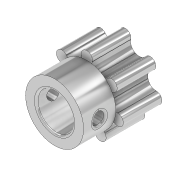
# Autodesk Inventor part: 4th Axis Drive Gears
Saved by Autodesk Inventor 2020 (Build 240168000, 168)
## iProperties
Created: 2021-06-27
Part Number: 4th Axis Drive Gears
Material: Generic
Document SubType Name: Modeling
Designer: Coy
Density: 1 g/cm^3
Appearance: Chrome - Polished
Author: Coy
Autodesk Inventor part; units mm, degrees
ref_plane "YZ Plane" through (0, 0, 0) normal (1, 0, 0) x (0, 1, 0)
ref_plane "XZ Plane" through (0, 0, 0) normal (0, 1, 0) x (-1, 0, 0)
ref_plane "XY Plane" through (0, 0, 0) normal (0, 0, 1) x (1, 0, 0)
sketch "Sketch1" plane through (0, 0, 0) normal (0, 0, 1) x (1, 0, 0)
  circle A0 centre (0, 0) radius 2.6
  circle A1 centre (0, 0) radius 6 construction
  line L0 (1.0268, 4.6361) -> (1.0416, 4.7025)
  line L1 (-1.0268, 4.6361) -> (-1.0416, 4.7025)
  line L2 (0, 0) -> (0, 12.6837) construction
  arc A2 (1.0416, 4.7025) -> (-1.0416, 4.7025) centre (0, 4.9332) ccw
  arc A3 (1.0268, 4.6361) -> (1.615, 3.4397) centre (2.0684, 4.4054) ccw
  arc A4 (-1.615, 3.4397) -> (-1.0268, 4.6361) centre (-2.0684, 4.4054) ccw
  arc A5 (-3.6962, 0.882) -> (-4.2649, 2.0877) centre (-4.7339, 1.1296) ccw
  arc A6 (-3.0272, 3.7463) -> (-4.326, 2.1176) centre (-3.8569, 3.0758) ccw
  arc A7 (-2.9844, 3.6934) -> (-1.6823, 3.4073) centre (-2.1546, 4.3639) ccw
  line L3 (-4.2649, 2.0877) -> (-4.326, 2.1176)
  line L4 (-2.9844, 3.6934) -> (-3.0272, 3.7463)
  arc A8 (-2.9941, -2.3399) -> (-4.2914, -2.0327) centre (-3.8347, -2.9968) ccw
  arc A9 (-4.8164, -0.031) -> (-4.3528, -2.0618) centre (-4.8095, -1.0977) ccw
  arc A10 (-4.7483, -0.0305) -> (-3.7129, 0.8091) centre (-4.7552, 1.0363) ccw
  line L5 (-4.2914, -2.0327) -> (-4.3528, -2.0618)
  line L6 (-4.7483, -0.0305) -> (-4.8164, -0.031)
  arc A11 (-0.0374, -3.7998) -> (-1.0864, -4.6225) centre (-0.0479, -4.8666) ccw
  arc A12 (-2.9788, -3.7849) -> (-1.1019, -4.6887) centre (-2.1404, -4.4447) ccw
  arc A13 (-2.9367, -3.7314) -> (-2.9475, -2.3984) centre (-3.775, -3.0717) ccw
  line L7 (-1.0864, -4.6225) -> (-1.1019, -4.6887)
  line L8 (-2.9367, -3.7314) -> (-2.9788, -3.7849)
  arc A14 (2.9475, -2.3984) -> (2.9367, -3.7314) centre (3.775, -3.0717) ccw
  arc A15 (1.1019, -4.6887) -> (2.9788, -3.7849) centre (2.1404, -4.4447) ccw
  arc A16 (1.0864, -4.6225) -> (0.0374, -3.7998) centre (0.0479, -4.8666) ccw
  line L9 (2.9367, -3.7314) -> (2.9788, -3.7849)
  line L10 (1.0864, -4.6225) -> (1.1019, -4.6887)
  arc A17 (3.7129, 0.8091) -> (4.7483, -0.0305) centre (4.7552, 1.0363) ccw
  arc A18 (4.3528, -2.0618) -> (4.8164, -0.031) centre (4.8095, -1.0977) ccw
  arc A19 (4.2914, -2.0327) -> (2.9941, -2.3399) centre (3.8347, -2.9968) ccw
  line L11 (4.7483, -0.0305) -> (4.8164, -0.031)
  line L12 (4.2914, -2.0327) -> (4.3528, -2.0618)
  arc A20 (1.6823, 3.4073) -> (2.9844, 3.6934) centre (2.1546, 4.3639) ccw
  arc A21 (4.326, 2.1176) -> (3.0272, 3.7463) centre (3.8569, 3.0758) ccw
  arc A22 (4.2649, 2.0877) -> (3.6962, 0.882) centre (4.7339, 1.1296) ccw
  line L13 (2.9844, 3.6934) -> (3.0272, 3.7463)
  line L14 (4.2649, 2.0877) -> (4.326, 2.1176)
  arc A23 (1.6823, 3.4073) -> (1.615, 3.4397) centre (0, 0) ccw
  arc A24 (3.7129, 0.8091) -> (3.6962, 0.882) centre (0, 0) ccw
  arc A25 (2.9475, -2.3984) -> (2.9941, -2.3399) centre (0, 0) ccw
  arc A26 (-0.0374, -3.7998) -> (0.0374, -3.7998) centre (0, 0) ccw
  arc A27 (-2.9941, -2.3399) -> (-2.9475, -2.3984) centre (0, 0) ccw
  arc A28 (-1.615, 3.4397) -> (-1.6823, 3.4073) centre (0, 0) ccw
  arc A29 (-3.6962, 0.882) -> (-3.7129, 0.8091) centre (0, 0) ccw
  line L15 (3.14, 3.5677) -> (3.1827, 3.6206)
  arc A30 (4.238, 2.2973) -> (3.1827, 3.6206) centre (3.8569, 3.0758) ccw
  line L16 (4.238, 2.2973) -> (4.1769, 2.2674)
  arc A31 (4.1769, 2.2674) -> (3.5017, 0.8356) centre (4.7339, 1.1296) ccw
  arc A32 (3.5174, 0.7665) -> (3.5017, 0.8356) centre (0, 0) ccw
  arc A33 (3.5174, 0.7665) -> (4.7471, -0.2305) centre (4.7552, 1.0363) ccw
  line L17 (4.7471, -0.2305) -> (4.8151, -0.231)
  arc A34 (4.4385, -1.8811) -> (4.8151, -0.231) centre (4.8095, -1.0977) ccw
  line L18 (4.4385, -1.8811) -> (4.377, -1.852)
  arc A35 (4.377, -1.852) -> (2.8365, -2.2168) centre (3.8347, -2.9968) ccw
  arc A36 (2.7924, -2.2721) -> (2.8365, -2.2168) centre (0, 0) ccw
  arc A37 (2.7924, -2.2721) -> (2.7795, -3.8551) centre (3.775, -3.0717) ccw
  line L19 (2.7795, -3.8551) -> (2.8216, -3.9086)
  arc A38 (1.2966, -4.643) -> (2.8216, -3.9086) centre (2.1404, -4.4447) ccw
  line L20 (1.2966, -4.643) -> (1.2811, -4.5767)
  arc A39 (1.2811, -4.5767) -> (0.0354, -3.5998) centre (0.0479, -4.8666) ccw
  arc A40 (-0.0354, -3.5998) -> (0.0354, -3.5998) centre (0, 0) ccw
  arc A41 (-0.0354, -3.5998) -> (-1.2811, -4.5767) centre (-0.0479, -4.8666) ccw
  line L21 (-1.2811, -4.5767) -> (-1.2966, -4.643)
  arc A42 (-2.8216, -3.9086) -> (-1.2966, -4.643) centre (-2.1404, -4.4447) ccw
  line L22 (-2.8216, -3.9086) -> (-2.7795, -3.8551)
  arc A43 (-2.7795, -3.8551) -> (-2.7924, -2.2721) centre (-3.775, -3.0717) ccw
  arc A44 (-2.8365, -2.2168) -> (-2.7924, -2.2721) centre (0, 0) ccw
  arc A45 (-2.8365, -2.2168) -> (-4.377, -1.852) centre (-3.8347, -2.9968) ccw
  line L23 (-4.377, -1.852) -> (-4.4385, -1.8811)
  arc A46 (-4.8151, -0.231) -> (-4.4385, -1.8811) centre (-4.8095, -1.0977) ccw
  line L24 (-4.8151, -0.231) -> (-4.7471, -0.2305)
  arc A47 (-4.7471, -0.2305) -> (-3.5174, 0.7665) centre (-4.7552, 1.0363) ccw
  arc A48 (-3.5017, 0.8356) -> (-3.5174, 0.7665) centre (0, 0) ccw
  arc A49 (-3.5017, 0.8356) -> (-4.1769, 2.2674) centre (-4.7339, 1.1296) ccw
  line L25 (-4.1769, 2.2674) -> (-4.238, 2.2973)
  arc A50 (-3.1827, 3.6206) -> (-4.238, 2.2973) centre (-3.8569, 3.0758) ccw
  line L26 (-3.1827, 3.6206) -> (-3.14, 3.5677)
  arc A51 (-3.14, 3.5677) -> (-1.5938, 3.228) centre (-2.1546, 4.3639) ccw
  arc A52 (-1.53, 3.2587) -> (-1.5938, 3.228) centre (0, 0) ccw
  arc A53 (-1.53, 3.2587) -> (-0.8316, 4.6793) centre (-2.0684, 4.4054) ccw
  line L27 (-0.8316, 4.6793) -> (-0.8463, 4.7458)
  arc A54 (0.8463, 4.7458) -> (-0.8463, 4.7458) centre (0, 4.9332) ccw
  line L28 (0.8463, 4.7458) -> (0.8316, 4.6793)
  arc A55 (0.8316, 4.6793) -> (1.53, 3.2587) centre (2.0684, 4.4054) ccw
  arc A56 (1.5938, 3.228) -> (1.53, 3.2587) centre (0, 0) ccw
  arc A57 (1.5938, 3.228) -> (3.14, 3.5677) centre (2.1546, 4.3639) ccw
  dimension "d0" = 5.2
  dimension "d1" = 12
  dimension "d5" = 2.1336
  dimension "d6" = 2.1336
  dimension "d7" = 2.1336
  dimension "d10" = 360
  dimension "d23" = 0.2
  constraints: 112 point on circle, 58 centre point, 58 end point, 5 tangent, 2 coincident, 2 line through centre, 1 point on line, 1 vertical, 140 other
  measures "d0" diameter of A0
  measures "d1" diameter of A1
  measures "d5" diameter of A2
  measures "d6" diameter of A3
  measures "d7" diameter of A4
  measures "d23" radial gap between concentric circles of A20 A57
extrude "Extrusion1" add sketch "Sketch1" against normal blind 6 contours L15 A30 L16 A31 A32 A33 L17 A34 L18 A35 A36 A37 L19 A38 L20 A39 A40 A41 L21 A42 L22 A43 A44 A45 L23 A46 L24 A47 A48 A49 L25 A50 L26 A51 A52 A53 L27 A54 L28 A55 A56 A57
sketch "Sketch2" plane through (0, 0, 0) normal (0, 0, 1) x (1, 0, 0)
  circle A0 centre (0, 0) radius 2.6 projected
  arc A1 (-1.615, 3.4397) -> (-1.6823, 3.4073) centre (0, 0) ccw projected
  circle A2 centre (0, 0) radius 3.8
  circle A3 centre (0, 0) radius 4.5
  point P0 (-1.6823, 3.4073)
  dimension "d24" = 9
  constraints: 2 coincident, 1 centre point, 3 other
  measures "d24" diameter of A3
extrude "Extrusion2" add sketch "Sketch2" along normal blind 5 contours A2 A1 | A3
sketch "Sketch3" plane through (0, 0, 0) normal (1, 0, 0) x (0, 1, 0)
  line L0 (3.8, 5) -> (-3.8, 5) projected
  line L1 (3.8, 5) -> (3.8, 0) projected
  line L2 (3.8, 2.5) -> (-3.8, 2.5) construction
  line L3 (-3.8, 5) -> (-3.8, -6) construction
  circle A0 centre (0, 2.5) radius 0.95
  point P0 (0, 0)
  dimension "d16" = 1.9
  constraints: 2 end point, 2 midpoint, 1 centre point, 1 horizontal, 1 point on line
  measures "d16" diameter of A0
extrude "Extrusion3" cut sketch "Sketch3" along normal through all both and the other way through all
chamfer "Chamfer1" distance 7 angle 2 1 edges at (-2.6, 0, 5) measured on face at (-2.6, 0, 4.5)
fillet "Fillet1" radius 0.3 5 edges at (-2.8444, 0, 5) (4.3986, -0.95, 2.5001) (4.4446, 0.7038, 3.1381) (4.4448, 0.703, 1.861) (-4.3986, -0.95, 2.5051)
equation "\"d6\" = d5"
equation "\"d7\" = d5"
body "Solid1"
